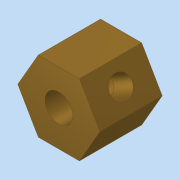
# Autodesk Inventor part: .125InchShaftHexNut
Saved by Autodesk Inventor 2017.3 (Build 213256000, 256)
## iProperties
Created: 2018-07-01
Part Number: .125InchShaftHexNut
Material: Brass, Soft Yellow
Document SubType Name: Modeling
Designer: Derek Wider
Density: 8.47 g/cm^3
Appearance: Brass - Satin
Author: Derek Wider
Autodesk Inventor part; units mm, degrees
ref_plane "YZ Plane" through (0, 0, 0) normal (1, 0, 0) x (0, 1, 0)
ref_plane "XZ Plane" through (0, 0, 0) normal (0, 1, 0) x (-1, 0, 0)
ref_plane "XY Plane" through (0, 0, 0) normal (0, 0, 1) x (1, 0, 0)
sketch "Sketch1" plane through (0, 0, 0) normal (0, 0, 1) x (1, 0, 0)
  circle A0 centre (0, 0) radius 1.5875
  line L0 (-4.6927, 0) -> (-2.3464, 4.064)
  line L1 (-2.3464, 4.064) -> (2.3464, 4.064)
  line L2 (2.3464, 4.064) -> (4.6927, 0)
  line L3 (4.6927, 0) -> (2.3464, -4.064)
  line L4 (2.3464, -4.064) -> (-2.3464, -4.064)
  line L5 (-2.3464, -4.064) -> (-4.6927, 0)
  dimension "d0" = 3.175
  dimension "d1" = 8.128
  constraints: 12 end point, 2 coincident, 1 centre point, 13 other
  measures "d0" diameter of A0
  measures "d1" distance between parallel lines of L4 L1
extrude "Extrusion1" add sketch "Sketch1" along normal blind 7.112
sketch "Sketch2" plane through (2.3464, 4.064, 7.112) normal (0.8660254, 0.5, 0) x (0, 0, -1)
  circle A0 centre (3.556, -2.3464) radius 1.27
  line L0 (0, -4.6927) -> (0, 0) projected
  line L1 (7.112, 0) -> (7.112, -4.6927) projected
  line L2 (7.112, 0) -> (0, 0) projected
  line L3 (0, -4.6927) -> (0, 0) projected
  line L4 (7.112, -4.6927) -> (0, -4.6927) projected
  line L5 (3.556, -2.3464) -> (3.556, 0) construction
  line L6 (7.112, 0) -> (0, 0) construction
  line L7 (3.556, -2.3464) -> (3.556, -4.6927) construction
  line L8 (7.112, -4.6927) -> (0, -4.6927) construction
  line L9 (3.556, -2.3464) -> (0, -2.3464) construction
  line L10 (3.556, -2.3464) -> (7.112, -2.3464) construction
  line L11 (7.112, -4.6927) -> (7.112, 0) construction
  dimension "d4" = 2.54
  constraints: 8 end point, 4 midpoint, 2 collinear, 2 perpendicular, 2 point on line, 1 centre point
  measures "d4" diameter of A0
extrude "Extrusion2" cut sketch "Sketch2" against normal up to next contours A0
body "Solid1"
